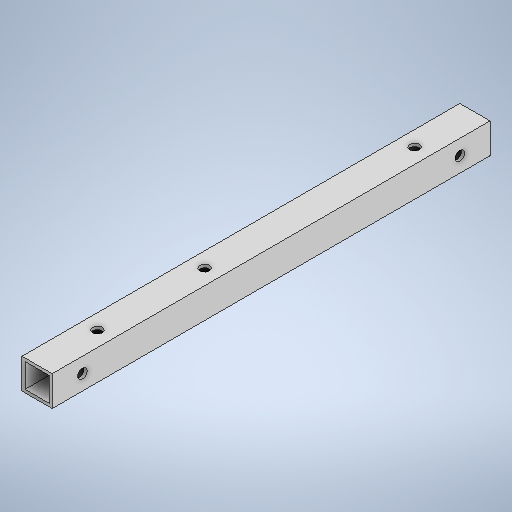
# Autodesk Inventor part: kaku_1010_plate
Saved by Autodesk Inventor 2025.1 (Build 291241000, 241)
## iProperties
Created: 2024-11-12
Part Number: kaku_1010_plate
Material: 一般
Document SubType Name: Modeling
Designer: yuki0520
Density: 1 g/cm^3
Appearance: 既定
Author: yuki0520
Autodesk Inventor part; units mm, degrees
ref_plane "YZ Plane" through (0, 0, 0) normal (1, 0, 0) x (0, 1, 0)
ref_plane "XZ Plane" through (0, 0, 0) normal (0, 1, 0) x (-1, 0, 0)
ref_plane "XY Plane" through (0, 0, 0) normal (0, 0, 1) x (1, 0, 0)
sketch "スケッチ1" plane through (0, 0, 0) normal (0, 0, 1) x (1, 0, 0)
  line L0 (5, -5) -> (-5, -5)
  line L1 (-5, -5) -> (-5, 5)
  line L2 (-5, 5) -> (5, 5)
  line L3 (5, 5) -> (5, -5)
  line L4 (5, -5) -> (-5, 5) construction
  line L5 (-5, -5) -> (5, 5) construction
  line L6 (4, 4) -> (-4, 4)
  line L7 (-4, 4) -> (-4, -4)
  line L8 (-4, -4) -> (4, -4)
  line L9 (4, -4) -> (4, 4)
  point P0 (0, 0)
  dimension "d0" = 10
  dimension "d1" = 10
  dimension "d2" = 1
  constraints: 20 end point, 4 parallel, 2 midpoint, 2 perpendicular, 1 horizontal, 3 other
  measures "d0" distance of L1.end L2.end
  measures "d1" distance of L0.end L1.end
  measures "d2" distance between parallel lines of L2 L6
extrude "押し出し1" add sketch "スケッチ1" along normal blind 145
sketch "スケッチ2" plane through (5, -5, 0) normal (1, 0, 0) x (0, 0, -1)
  line L0 (0, 5) -> (-145, 5)
  line L1 (0, 1) -> (-145, 1) projected
  line L2 (0, 0) -> (0, 10) projected
  point P0 (-135, 5)
  point P1 (-10, 5)
  dimension "d5" = 10
  dimension "d6" = 125
  constraints: 2 end point, 2 point on line, 1 parallel
  measures "d5" distance from line of L2 point (-10, 5)
  measures "d6" distance of point (-135, 5) point (-10, 5)
hole "穴1" at (5, 0, 135) at (5, 0, 10) direction (-1, 0, 0) diameter 3.2 end through all
sketch "スケッチ3" plane through (-5, 5, 0) normal (0, 1, 0) x (1, 0, 0)
  line L0 (5, 0) -> (5, -145)
  line L1 (10, -145) -> (0, -145) projected
  line L2 (10, 0) -> (0, 0) projected
  point P0 (5, -125)
  point P1 (5, -20)
  point P2 (5, -89.5)
  point P3 (5, -72.5)
  dimension "d14" = 20
  dimension "d15" = 105
  dimension "d24" = 17
  dimension "d25" = 89.5
  constraints: 3 point on line, 2 end point, 2 midpoint
  measures "d14" distance from line of L2 point (5, -20)
  measures "d15" distance of point (5, -125) point (5, -20)
  measures "d24" distance of point (5, -72.5) point (5, -89.5)
  measures "d25" distance from line of L2 point (5, -89.5)
hole "穴2" at (0, 5, 125) at (0, 5, 20) at (0, 5, 89.5) direction (0, -1, 0) diameter 3.2 end through all
